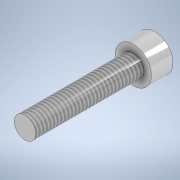
# Autodesk Inventor part: tornilloM6x30mm
Saved by Autodesk Inventor 2021.5 (Build 255421000, 421)
## iProperties
Created: 2024-11-29
Part Number: tornilloM6x30mm
Material: Aluminio 6061-AHC
Document SubType Name: Modeling
Designer: Joho_
Mass: 3.31003 g
Surface Area: 9.83062 cm^2
Volume: 1.22594 cm^3
Density: 2.7 g/cm^3
Appearance: Aluminio - Oscuro
Author: Joho_
Autodesk Inventor part; units mm, degrees
ref_plane "YZ Plane" through (0, 0, 0) normal (1, 0, 0) x (0, 1, 0)
ref_plane "XZ Plane" through (0, 0, 0) normal (0, 1, 0) x (-1, 0, 0)
ref_plane "XY Plane" through (0, 0, 0) normal (0, 0, 1) x (1, 0, 0)
sketch "Boceto1" plane through (0, 0, 0) normal (0, 0, 1) x (1, 0, 0)
  circle A0 centre (0, 0) radius 3
  circle A1 centre (0, 0) radius 5
  dimension "d0" = 6
  dimension "d1" = 10
  constraints: 3 coincident, 2 centre point
  measures "d0" diameter of A0
  measures "d1" diameter of A1
extrude "Extrusión1" add sketch "Boceto1" along normal blind 30 contours A0
extrude "Extrusión2" add sketch "Boceto1" against normal blind 6 contours A0 | A1
thread "Rosca1" size "M6x1" class "6g" standard "ANSI Metric M Profile" full length
sketch "Boceto2" plane through (0, 0, -6) normal (0, 0, -1) x (-1, 0, 0)
  line L0 (3, 0) -> (1.5, -2.5981)
  line L1 (1.5, -2.5981) -> (-1.5, -2.5981)
  line L2 (-1.5, -2.5981) -> (-3, 0)
  line L3 (-3, 0) -> (-1.5, 2.5981)
  line L4 (-1.5, 2.5981) -> (1.5, 2.5981)
  line L5 (1.5, 2.5981) -> (3, 0)
  point P0 (0, 0)
  point P1 (0, 0)
  dimension "d8" = 6
  constraints: 12 end point, 1 coincident, 13 other
  measures "d8" distance of L0.start L2.end
extrude "Extrusión3" cut sketch "Boceto2" against normal blind 4
